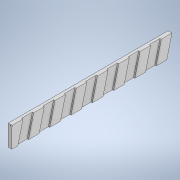
# Autodesk Inventor part: box hole filler
Saved by Autodesk Inventor 2021 (Build 250183000, 183)
## iProperties
Created: 2021-06-29
Part Number: box hole filler
Material: Generic
Document SubType Name: Modeling
Designer: newic
Density: 1 g/cm^3
Appearance: Default
Author: newic
Autodesk Inventor part; units mm, degrees
ref_plane "YZ Plane" through (0, 0, 0) normal (1, 0, 0) x (0, 1, 0)
ref_plane "XZ Plane" through (0, 0, 0) normal (0, 1, 0) x (-1, 0, 0)
ref_plane "XY Plane" through (0, 0, 0) normal (0, 0, 1) x (1, 0, 0)
sketch "Sketch1" plane through (0, 0, 0) normal (1, 0, 0) x (0, 1, 0)
  line L0 (0, 0) -> (25.4, 0)
  line L1 (0, 0) -> (0, -190.5)
  line L2 (25.4, 0) -> (25.4, -196.85)
  line L3 (25.4, -196.85) -> (0, -190.5)
  dimension "d0" = 25.4
  dimension "d1" = 190.5
  dimension "d2" = 196.85
  constraints: 8 end point, 2 vertical, 1 horizontal
  measures "d0" distance of L0.start L0.end
  measures "d1" distance of L0.start L1.end
  measures "d2" distance of L0.end L2.end
extrude "Extrusion1" add sketch "Sketch1" along normal blind 3.175
sketch "Sketch2" plane through (3.175, 0, 0) normal (1, 0, 0) x (0, 0, -1)
  line L0 (190.5, 0) -> (196.85, 25.4) projected
  line L1 (196.85, 25.4) -> (0, 25.4) projected
  line L2 (0, 25.4) -> (0, 0) projected
  line L3 (0, 0) -> (190.5, 0) projected
  line L4 (0, 0) -> (190.5, 0) projected
  line L5 (190.5, 0) -> (196.85, 25.4) projected
  line L6 (128.1187, -249.5251) -> (257.6151, 268.4604)
  line L7 (115.7979, -246.4449) -> (245.2943, 271.5406)
  line L8 (103.4771, -243.3647) -> (232.9735, 274.6208)
  line L9 (91.1563, -240.2845) -> (220.6527, 277.701)
  line L10 (78.8355, -237.2043) -> (208.3319, 280.7812)
  line L11 (66.5147, -234.1241) -> (196.011, 283.8614)
  line L12 (54.1939, -231.0439) -> (183.6902, 286.9416)
  line L13 (41.8731, -227.9637) -> (171.3694, 290.0218)
  line L14 (29.5522, -224.8835) -> (159.0486, 293.102)
  line L15 (17.2314, -221.8033) -> (146.7278, 296.1822)
  line L16 (4.9106, -218.7231) -> (134.407, 299.2624)
  line L17 (-7.4102, -215.6429) -> (122.0862, 302.3426)
  line L18 (-19.731, -212.5627) -> (109.7654, 305.4228)
  line L19 (-32.0518, -209.4825) -> (97.4446, 308.503)
  line L20 (-44.3726, -206.4023) -> (85.1238, 311.5832)
  line L21 (-56.6934, -203.3221) -> (72.8029, 314.6634)
  point P0 (183.7591, 25.4)
  point P1 (177.4091, 0)
  point P2 (157.5774, 25.4)
  point P3 (151.2274, 0)
  point P4 (164.3183, 0)
  point P5 (170.6683, 25.4)
  point P6 (131.3957, 25.4)
  point P7 (125.0457, 0)
  point P8 (138.1366, 0)
  point P9 (144.4866, 25.4)
  point P10 (105.214, 25.4)
  point P11 (98.864, 0)
  point P12 (111.9548, 0)
  point P13 (118.3048, 25.4)
  point P14 (79.0323, 25.4)
  point P15 (72.6823, 0)
  point P16 (85.7731, 0)
  point P17 (92.1231, 25.4)
  point P18 (52.8505, 25.4)
  point P19 (46.5005, 0)
  point P20 (59.5914, 0)
  point P21 (65.9414, 25.4)
  point P22 (26.6688, 25.4)
  point P23 (20.3188, 0)
  point P24 (33.4097, 0)
  point P25 (39.7597, 25.4)
  point P26 (0.4871, 25.4)
  point P27 (0, 23.4516)
  point P28 (7.228, 0)
  point P29 (13.578, 25.4)
  dimension "d7" = 12.7
  dimension "d8" = 12.7
  dimension "d9" = 12.7
  dimension "d10" = 12.7
  dimension "d11" = 12.7
  dimension "d12" = 12.7
  dimension "d13" = 12.7
  dimension "d14" = 12.7
  dimension "d15" = 12.7
  dimension "d16" = 12.7
  dimension "d17" = 12.7
  dimension "d18" = 12.7
  dimension "d19" = 12.7
  dimension "d20" = 12.7
  dimension "d21" = 12.7
  constraints: 32 end point, 15 parallel
  measures "d7" distance between parallel lines of L6 L7
  measures "d8" distance between parallel lines of L7 L8
  measures "d9" distance between parallel lines of L8 L9
  measures "d10" distance between parallel lines of L9 L10
  measures "d11" distance between parallel lines of L10 L11
  measures "d12" distance between parallel lines of L11 L12
  measures "d13" distance between parallel lines of L12 L13
  measures "d14" distance between parallel lines of L13 L14
  measures "d15" distance between parallel lines of L14 L15
  measures "d16" distance between parallel lines of L15 L16
  measures "d17" distance between parallel lines of L16 L17
  measures "d18" distance between parallel lines of L17 L18
  measures "d19" distance between parallel lines of L18 L19
  measures "d20" distance between parallel lines of L19 L20
  measures "d21" distance between parallel lines of L20 L21
extrude "Extrusion2" add sketch "Sketch2" along normal blind 1.5875 contours L3 L7 L1 L0 | L3 L9 L1 L8 | L3 L11 L1 L10 | L3 L13 L1 L12 | L3 L15 L1 L14 | L3 L17 L1 L16 | L3 L19 L1 L18 | L3 L2 L21 L1 L20
body "Solid1"
